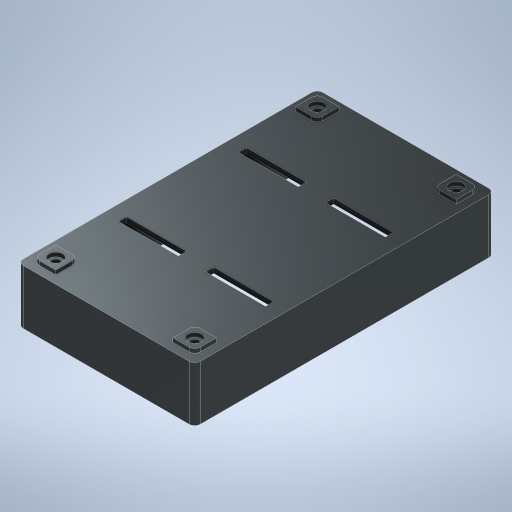
# Autodesk Inventor part: Part 2 edit
Saved by Autodesk Inventor 2023 (Build 270158000, 158)
## iProperties
Created: 2023-03-26
Part Number: Part 2 edit
Material: Generic
Document SubType Name: Modeling
Designer: IanJm
Density: 1 g/cm^3
Appearance: Iron Gray
Author: IanJm
Autodesk Inventor part; units mm, degrees
ref_plane "YZ Plane" through (0, 0, 0) normal (1, 0, 0) x (0, 1, 0)
ref_plane "XZ Plane" through (0, 0, 0) normal (0, 1, 0) x (-1, 0, 0)
ref_plane "XY Plane" through (0, 0, 0) normal (0, 0, 1) x (1, 0, 0)
sketch "Sketch1" plane through (0, 0, 0) normal (0, 1, 0) x (-1, 0, 0)
  line L0 (0, -2) -> (0, -108)
  line L1 (2, -110) -> (63, -110)
  line L2 (2, 0) -> (63, 0)
  line L3 (65, -2) -> (65, -108)
  line L4 (0, 0) -> (0, -3)
  line L5 (65, 0) -> (57, 0)
  line L6 (0, -110) -> (0, -107)
  line L7 (0, 0) -> (3, 0)
  arc A0 (65, -2) -> (63, 0) centre (63, -2) ccw
  arc A1 (2, 0) -> (0, -2) centre (2, -2) ccw
  arc A2 (0, -108) -> (2, -110) centre (2, -108) ccw
  arc A3 (63, -110) -> (65, -108) centre (63, -108) ccw
  arc A4 (5, -3) -> (3, -5) centre (5, -5) ccw
  circle A5 centre (7, -7) radius 1.5
  line L8 (11, -3) -> (11, -9)
  line L9 (9, -11) -> (3, -11)
  arc A6 (9, -11) -> (11, -9) centre (9, -9) ccw
  line L10 (3, -5) -> (3, -11)
  arc A7 (3, -105) -> (5, -107) centre (5, -105) ccw
  circle A8 centre (7, -103) radius 1.5
  line L11 (11, -107) -> (11, -101)
  line L12 (9, -99) -> (3, -99)
  arc A9 (11, -101) -> (9, -99) centre (9, -101) ccw
  line L13 (3, -105) -> (3, -99)
  line L14 (3, -11) -> (3, -99)
  line L15 (11, -107) -> (5, -107)
  line L16 (11, -3) -> (5, -3)
  arc A10 (62, -5) -> (60, -3) centre (60, -5) ccw
  circle A11 centre (58, -7) radius 1.5
  line L17 (54, -3) -> (54, -9)
  line L18 (56, -11) -> (62, -11)
  arc A12 (54, -9) -> (56, -11) centre (56, -9) ccw
  line L19 (62, -5) -> (62, -11)
  arc A13 (56, -99) -> (54, -101) centre (56, -101) ccw
  circle A14 centre (58, -103) radius 1.5
  line L20 (56, -99) -> (62, -99)
  line L21 (62, -105) -> (62, -99)
  arc A15 (60, -107) -> (62, -105) centre (60, -105) ccw
  line L22 (54, -107) -> (54, -101)
  line L23 (62, -11) -> (62, -99)
  line L24 (54, -107) -> (60, -107)
  line L25 (54, -3) -> (60, -3)
  line L26 (54, -107) -> (11, -107)
  line L27 (54, -3) -> (11, -3)
  point P0 (65, -110)
  point P1 (55, -5)
  point P2 (55, -105)
  dimension "d0" = 110
  dimension "d1" = 65
  dimension "d2" = 3
  dimension "d4" = 3
  dimension "d5" = 3
  dimension "d8" = 2
  constraints: 56 end point, 24 point on circle, 16 centre point, 12 point on line, 10 tangent, 4 equal radius, 3 perpendicular, 2 horizontal, 2 parallel, 2 vertical, 1 collinear
  measures "d0" distance of L4.start L6.start
  measures "d1" distance of L6.start point (65, -110)
  measures "d2" distance of L4.start L4.end
  measures "d4" distance of L6.start L6.end
  measures "d5" distance of L4.start L7.end
  measures "d8" radius of A0
extrude "Extrusion18" add sketch "Sketch1" along normal blind 20 contours A1 L2 A0 L3 A3 L1 A2 L0 | L16 L8 A6 L9 L10 A4 | L27 L17 A12 L18 L23 L20 A13 L22 L26 L11 A9 L12 L14 L9 A6 L8 | L25 A10 L19 L18 A12 L17 | L12 A9 L11 L15 A7 L13 | L21 A15 L24 L22 A13 L20 | A5 | A8 | A11 | A14
extrude "Extrusion19" cut sketch "Sketch1" along normal blind 18 contours L27 L17 A12 L18 L23 L20 A13 L22 L26 L11 A9 L12 L14 L9 A6 L8
extrude "Extrusion20" cut sketch "Sketch1" along normal blind 20 contours A5 | A8 | A11 | A14
extrude "Extrusion21" add sketch "Sketch1" along normal blind 21.5 contours L16 L8 A6 L9 L10 A4 | L25 A10 L19 L18 A12 L17 | L12 A9 L11 L15 A7 L13 | L21 A15 L24 L22 A13 L20
sketch "Sketch11" plane through (0, 21.5, 0) normal (0, 1, 0) x (1, 0, 0)
  circle A0 centre (-7, 7) radius 1.5 projected
  circle A1 centre (-7, 7) radius 2.5
  circle A2 centre (-7, 103) radius 1.5 projected
  circle A3 centre (-7, 103) radius 2.5
  circle A4 centre (-58, 103) radius 1.5 projected
  circle A5 centre (-58, 103) radius 2.5
  circle A6 centre (-58, 7) radius 1.5 projected
  circle A7 centre (-58, 7) radius 2.5
  point P0 (0, 0)
  dimension "d166" = 5
  dimension "d167" = 5
  dimension "d168" = 5
  dimension "d169" = 5
  constraints: 4 centre point, 4 coincident
  measures "d166" diameter of A1
  measures "d167" diameter of A3
  measures "d168" diameter of A5
  measures "d169" diameter of A7
extrude "Extrusion22" cut sketch "Sketch11" against normal blind 1.5 contours A1 | A3 | A5 | A6 | A7
sketch "Sketch12" plane through (-65, 0, -108) normal (-1, 0, 0) x (0, 0, 1)
  line L0 (99, 0) -> (99, 18) projected
  line L1 (7, 0) -> (7, 18) projected
  line L2 (99, 0) -> (7, 0)
  line L3 (97, 0) -> (9, 0) projected
  line L4 (53, 2) -> (27, 2)
  line L5 (53, 2) -> (79, 2)
  line L6 (80, 1) -> (80, 0)
  line L7 (26, 1) -> (26, 0)
  line L8 (20, 10) -> (14, 10)
  line L9 (13, 11) -> (13, 11.5)
  line L10 (21, 11) -> (21, 11.5)
  line L11 (20, 12.5) -> (14, 12.5)
  arc A0 (80, 1) -> (79, 2) centre (79, 1) ccw
  arc A1 (27, 2) -> (26, 1) centre (27, 1) ccw
  arc A2 (20, 10) -> (21, 11) centre (20, 11) ccw
  arc A3 (21, 11.5) -> (20, 12.5) centre (20, 11.5) ccw
  arc A4 (14, 12.5) -> (13, 11.5) centre (14, 11.5) ccw
  arc A5 (13, 11) -> (14, 10) centre (14, 11) ccw
  point P0 (108, 0)
  point P1 (26, 2)
  point P2 (80, 2)
  point P3 (21, 10)
  point P4 (13, 10)
  point P5 (13, 12.5)
  dimension "d173" = 27
  dimension "d174" = 27
  dimension "d179" = 8
  dimension "d180" = 2.5
  dimension "d181" = 1
  dimension "d182" = 1
  constraints: 18 end point, 12 point on circle, 12 point on line, 12 tangent, 6 centre point, 5 perpendicular, 4 equal radius, 2 horizontal, 1 vertical
  measures "d173" distance of L4.start point (26, 2)
  measures "d174" distance of L4.start point (80, 2)
  measures "d179" distance of point (21, 10) point (13, 10)
  measures "d180" distance of point (13, 10) point (13, 12.5)
  measures "d181" radius of A0
  measures "d182" radius of A2
extrude "Extrusion23" cut sketch "Sketch12" against normal blind 3
sketch "Sketch13" plane through (0, 20, 0) normal (0, 1, 0) x (1, 0, 0)
  line L0 (-62, 11) -> (-56, 11) projected
  line L1 (-3, 99) -> (-9, 99) projected
  line L2 (-62, 99) -> (-3, 99)
  line L3 (-3, 11) -> (-3, 99) projected
  line L4 (-3, 99) -> (-3, 11)
  line L5 (-3, 11) -> (-62, 11)
  line L6 (-62, 55) -> (-3, 55)
  line L7 (-62, 55) -> (-62, 11)
  line L8 (-62, 29) -> (-62, 81) projected
  line L9 (-3, 55) -> (-62, 55)
  line L10 (-37.5, 34.5) -> (-59.5, 34.5)
  line L11 (-59.5, 34.5) -> (-59.5, 31.5)
  line L12 (-59.5, 31.5) -> (-37.5, 31.5)
  line L13 (-37.5, 31.5) -> (-37.5, 34.5)
  line L14 (-27.5, 34.5) -> (-5.5, 34.5)
  line L15 (-5.5, 34.5) -> (-5.5, 31.5)
  line L16 (-5.5, 31.5) -> (-27.5, 31.5)
  line L17 (-27.5, 31.5) -> (-27.5, 34.5)
  line L18 (-37.5, 75.5) -> (-59.5, 75.5)
  line L19 (-59.5, 75.5) -> (-59.5, 78.5)
  line L20 (-59.5, 78.5) -> (-37.5, 78.5)
  line L21 (-37.5, 78.5) -> (-37.5, 75.5)
  line L22 (-27.5, 75.5) -> (-5.5, 75.5)
  line L23 (-5.5, 75.5) -> (-5.5, 78.5)
  line L24 (-5.5, 78.5) -> (-27.5, 78.5)
  line L25 (-27.5, 78.5) -> (-27.5, 75.5)
  point P0 (0, 0)
  dimension "d202" = 22
  dimension "d203" = 3
  constraints: 44 end point, 8 symmetric about line, 4 perpendicular, 1 collinear, 1 horizontal, 1 midpoint, 1 vertical
  measures "d202" distance of L10.start L10.end
  measures "d203" distance of L10.end L11.end
extrude "Extrusion24" cut sketch "Sketch13" against normal blind 3 contours L13 L12 L11 L10 | L14 L15 L16 L17 | L18 L19 L20 L21 | L25 L24 L23 L22
sketch "Sketch14" plane through (-2, 0, -110) normal (0, 0, -1) x (-1, 0, 0)
  line L0 (0, 0) -> (61, 0) projected
  line L1 (7, 0) -> (7, 18) projected
  line L2 (13.5993, 5.8762) -> (13.5993, 13.8762)
  line L3 (14.5993, 14.8762) -> (32.5993, 14.8762)
  line L4 (33.5993, 13.8762) -> (33.5993, 5.8762)
  line L5 (32.5993, 4.8762) -> (14.5993, 4.8762)
  arc A0 (32.5993, 4.8762) -> (33.5993, 5.8762) centre (32.5993, 5.8762) ccw
  arc A1 (13.5993, 5.8762) -> (14.5993, 4.8762) centre (14.5993, 5.8762) ccw
  arc A2 (14.5993, 14.8762) -> (13.5993, 13.8762) centre (14.5993, 13.8762) ccw
  arc A3 (33.5993, 13.8762) -> (32.5993, 14.8762) centre (32.5993, 13.8762) ccw
  point P0 (-2, 0)
  point P1 (13.5993, 4.8762)
  point P2 (13.5993, 14.8762)
  point P3 (33.5993, 14.8762)
  dimension "d194" = 10
  dimension "d195" = 20
  dimension "d196" = 1
  constraints: 8 end point, 8 point on circle, 8 tangent, 6 point on line, 4 centre point, 3 equal radius, 3 perpendicular, 1 vertical
  measures "d194" distance of point (13.599, 4.876) point (13.599, 14.876)
  measures "d195" distance of point (13.599, 14.876) point (33.599, 14.876)
  measures "d196" radius of A0
extrude "Extrusion25" cut sketch "Sketch14" against normal blind 3
body "Solid3"
